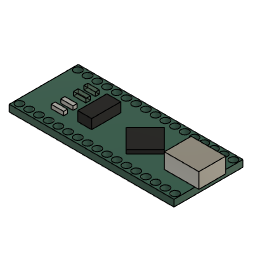
vacuum_box (Autodesk Fusion 360 archive; units mm, degrees)
design "arduino_nano"
Autodesk Fusion 360 part; units mm, degrees
sketch "Sketch1" plane through (0, 0, 0) normal (0, 0, 1) x (1, 0, 0)
  line L0 (21.5, 9) -> (-21.5, 9)
  line L1 (-21.5, 9) -> (-21.5, -9)
  line L2 (-21.5, -9) -> (21.5, -9)
  line L3 (21.5, -9) -> (21.5, 9)
  line L4 (21.5, 9) -> (-21.5, -9) construction
  line L5 (-21.5, 9) -> (21.5, -9) construction
  line L6 (13.5, 3.5) -> (22.5, 3.5)
  line L7 (22.5, 3.5) -> (22.5, -3.5)
  line L8 (22.5, -3.5) -> (13.5, -3.5)
  line L9 (13.5, -3.5) -> (13.5, 3.5)
  line L10 (13.5, 3.5) -> (22.5, -3.5) construction
  line L11 (22.5, 3.5) -> (13.5, -3.5) construction
  circle A0 centre (-20.3, 7.7) radius 1
  circle A1 centre (-17.76, 7.7) radius 1
  circle A2 centre (-15.22, 7.7) radius 1
  circle A3 centre (-12.68, 7.7) radius 1
  circle A4 centre (-10.14, 7.7) radius 1
  circle A5 centre (-7.6, 7.7) radius 1
  circle A6 centre (-5.06, 7.7) radius 1
  circle A7 centre (-2.52, 7.7) radius 1
  circle A8 centre (0.02, 7.7) radius 1
  circle A9 centre (2.56, 7.7) radius 1
  circle A10 centre (5.1, 7.7) radius 1
  circle A11 centre (7.64, 7.7) radius 1
  circle A12 centre (10.18, 7.7) radius 1
  circle A13 centre (12.72, 7.7) radius 1
  circle A14 centre (15.26, 7.7) radius 1
  circle A15 centre (17.8, 7.7) radius 1
  circle A16 centre (20.34, 7.7) radius 1
  circle A17 centre (10.18, -7.54) radius 1
  circle A18 centre (-7.6, -7.54) radius 1
  circle A19 centre (17.8, -7.54) radius 1
  circle A20 centre (-15.22, -7.54) radius 1
  circle A21 centre (2.56, -7.54) radius 1
  circle A22 centre (0.02, -7.54) radius 1
  circle A23 centre (5.1, -7.54) radius 1
  circle A24 centre (-10.14, -7.54) radius 1
  circle A25 centre (7.64, -7.54) radius 1
  circle A26 centre (-2.52, -7.54) radius 1
  circle A27 centre (-5.06, -7.54) radius 1
  circle A28 centre (-12.68, -7.54) radius 1
  circle A29 centre (-20.3, -7.54) radius 1
  circle A30 centre (15.26, -7.54) radius 1
  circle A31 centre (20.34, -7.54) radius 1
  circle A32 centre (12.72, -7.54) radius 1
  circle A33 centre (-17.76, -7.54) radius 1
  line L12 (5, 5) -> (10, 0)
  line L13 (10, 0) -> (5, -5)
  line L14 (5, 5) -> (0, 0)
  line L15 (0, 0) -> (5, -5)
  line L16 (-8.6108, 3.6045) -> (-5, 3.6045)
  line L17 (-5, 3.6045) -> (-5, -4)
  line L18 (-5, -4) -> (-8.6108, -4)
  line L19 (-8.6108, -4) -> (-8.6108, 3.6045)
  line L20 (-15, 5) -> (-12, 5)
  line L21 (-12, 5) -> (-12, 4)
  line L22 (-12, 4) -> (-15, 4)
  line L23 (-15, 4) -> (-15, 5)
  line L24 (-15, 2.5) -> (-11.7833, 2.5)
  line L25 (-11.7833, 2.5) -> (-11.7833, 1.2848)
  line L26 (-11.7833, 1.2848) -> (-15, 1.2848)
  line L27 (-15, 1.2848) -> (-15, 2.5)
  line L28 (-15, -1) -> (-11.7833, -1)
  line L29 (-11.7833, -1) -> (-11.7833, -2.0626)
  line L30 (-11.7833, -2.0626) -> (-15, -2.0626)
  line L31 (-15, -2.0626) -> (-15, -1)
  line L32 (-15, -3.5) -> (-11.7833, -3.5)
  line L33 (-11.7833, -3.5) -> (-11.7833, -4.5258)
  line L34 (-11.7833, -4.5258) -> (-15, -4.5258)
  line L35 (-15, -4.5258) -> (-15, -3.5)
  point P0 (18, 0)
  dimension "d1" = 43
  dimension "d2" = 18
  dimension "d3" = 9
  dimension "d4" = 7
  dimension "d5" = 2
  dimension "d8" = 2.54
  dimension "d9" = 0
  dimension "d12" = 2.54
  dimension "d13" = 0
  dimension "d14" = 2
  constraint horizontal L0
  constraint perpendicular L0 L1
  constraint parallel L0 L2
  constraint parallel L1 L3
  constraint coincident L4 L14.end
  constraint coincident L5 L14.end
  constraint coincident L14.end L15.start
  constraint horizontal L6
  constraint perpendicular L6 L7
  constraint parallel L6 L8
  constraint parallel L7 L9
  constraint coincident L10 P0
  constraint coincident L11 P0
  constraint perpendicular L12 L13
  constraint perpendicular L12 L14
  constraint perpendicular L13 L15
  constraint horizontal L16
  constraint vertical L17
  constraint horizontal L18
  constraint vertical L19
  constraint coincident L5 L16.start
  constraint horizontal L20
  constraint vertical L21
  constraint horizontal L22
  constraint vertical L23
  constraint horizontal L24
  constraint vertical L25
  constraint horizontal L26
  constraint vertical L27
  constraint horizontal L28
  constraint vertical L29
  constraint horizontal L30
  constraint vertical L31
  constraint horizontal L32
  constraint vertical L33
  constraint horizontal L34
  constraint vertical L35
  measures "d1" distance of L1.end L2.end
  measures "d2" distance of L0.end L1.end
  measures "d3" distance of L7.end L8.end
  measures "d4" distance of L6.end L7.end
  measures "d5" diameter of A0
  measures "d14" diameter of A29
extrude "Extrude1" add sketch "Sketch1" against normal blind 1.75 contours L0 L1 L2 L3 L6 L8 L9 | L3 L6 L8 L9 | L12 L13 L14 L15 | L16 L17 L18 L19 | L20 L21 L22 L23 | L24 L25 L26 L27 | L28 L29 L30 L31 | L32 L33 L34 L35 makes body 1
extrude "Extrude2" add sketch "Sketch1" along normal blind 1 separate body contours L12 L13 L14 L15 | L20 L21 L22 L23 | L24 L25 L26 L27 | L28 L29 L30 L31 | L32 L33 L34 L35 makes body 2 at (-13.9278, -1.3542, 0) makes body 3 at (-13.9278, 2.0949, 0) makes body 4 at (-13.9278, -3.8419, 0) makes body 5 at (-14, 4.6667, 0) makes body 6 at (5, 1.6667, 0)
extrude "Extrude3" add sketch "Sketch1" along normal blind 2.5 separate body contours L16 L17 L18 L19 makes body 7
extrude "Extrude4" add sketch "Sketch1" along normal blind 4 separate body contours L3 L6 L7 L8 | L3 L6 L8 L9 makes body 8
